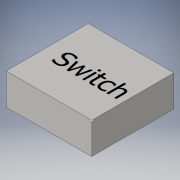
# Autodesk Inventor part: switch-ver1-1111-2017
Saved by Autodesk Inventor 2016 SP1 (Build 200210100, 210)
## iProperties
Created: 2017-02-08
Part Number: switch-ver1-1111-2017
Material: Generic
Document SubType Name: Modeling
Designer: 601898
Density: 1 g/cm^3
Appearance: Default
Author: 601898
Autodesk Inventor part; units mm, degrees
ref_plane "YZ Plane" through (0, 0, 0) normal (1, 0, 0) x (0, 1, 0)
ref_plane "XZ Plane" through (0, 0, 0) normal (0, 1, 0) x (-1, 0, 0)
ref_plane "XY Plane" through (0, 0, 0) normal (0, 0, 1) x (1, 0, 0)
sketch "Sketch1" plane through (0, 0, 0) normal (0, 1, 0) x (-1, 0, 0)
  line L0 (0, 0) -> (101.092, 0)
  line L1 (101.092, 0) -> (101.092, -97.1042)
  line L2 (101.092, -97.1042) -> (0, -97.1042)
  line L3 (0, -97.1042) -> (0, 0)
  dimension "d0" = 101.092
  dimension "d1" = 97.1042
  constraints: 8 end point, 2 parallel, 1 horizontal, 1 perpendicular
  measures "d0" distance of L1.end L2.end
  measures "d1" distance of L0.end L1.end
extrude "Extrusion1" add sketch "Sketch1" along normal blind 37.084
sketch "Sketch2" plane through (0, 37.084, 0) normal (0, 1, 0) x (1, 0, 0)
  line L0 (-86.0168, 57.6178) -> (-24.7466, 57.6178) construction
  line L1 (-24.7466, 57.6178) -> (-24.7466, 30.9333) construction
  line L2 (-24.7466, 30.9333) -> (-86.0168, 30.9333) construction
  line L3 (-86.0168, 30.9333) -> (-86.0168, 57.6178) construction
  point P0 (0, 0)
  constraints: 2 other
body "Solid1"
